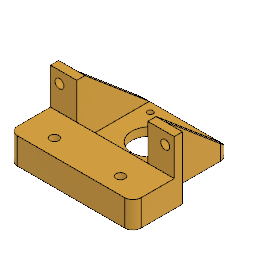
new2_elevated_Z_Motor_Mount v15 (Autodesk Fusion 360 design; units mm, degrees)
Autodesk Fusion 360 part; units mm, degrees
sketch "Sketch14" plane through (0, 0, 0) normal (0, 0, 1) x (1, 0, 0)
  line L0 (-37.5, 21) -> (37.5, 21)
  line L1 (37.5, 21) -> (37.5, -48)
  line L2 (37.5, -48) -> (-37.5, -48)
  line L3 (-37.5, -48) -> (-37.5, 21)
  line L4 (0, 21) -> (0, -48) construction
  circle A0 centre (0, 0) radius 11.2
  line L5 (15.5, 15.5) -> (-15.5, 15.5) construction
  line L6 (-15.5, 15.5) -> (-15.5, -15.5) construction
  line L7 (-15.5, -15.5) -> (15.5, -15.5) construction
  line L8 (15.5, -15.5) -> (15.5, 15.5) construction
  line L9 (15.5, 15.5) -> (-15.5, -15.5) construction
  line L10 (-15.5, 15.5) -> (15.5, -15.5) construction
  circle A1 centre (15.5, -15.5) radius 1.7
  circle A2 centre (15.5, 15.5) radius 1.7
  line L11 (-37.5, -38) -> (37.5, -38) construction
  circle A3 centre (20, -38) radius 5.5
  line L12 (26.5, 21) -> (26.5, -18)
  line L13 (26.5, -18) -> (37.5, -18)
  line L14 (-26.5, 21) -> (-26.5, -18)
  line L15 (-26.5, -18) -> (-37.5, -18)
  circle A4 centre (-20, -38) radius 5.5
  circle A5 centre (-15.5, 15.5) radius 1.7
  circle A6 centre (-15.5, -15.5) radius 1.7
  line L16 (-26.5, -18) -> (26.5, -18)
  line L17 (-37.5, -23) -> (37.5, -23)
  line L18 (21.5, 21) -> (21.5, -18)
  line L19 (-21.5, 21) -> (-21.5, -18)
  circle A7 centre (20, -38) radius 2.7
  circle A8 centre (-20, -38) radius 2.7
  line L20 (21.5, -18) -> (21.5, -23)
  line L21 (-21.5, -18) -> (-21.5, -23)
  dimension "d71" = 75
  dimension "d72" = 21
  dimension "d73" = 22.4
  dimension "d76" = 3.4
  dimension "d77" = 3.4
  dimension "d81" = 11
  dimension "d82" = 10
  dimension "d84" = 20
  dimension "d85" = 11
  dimension "d87" = 5
  dimension "d88" = 5
  dimension "d89" = 5.4
  dimension "d121" = 18
  dimension "d123" = 15
  dimension "d126" = 15.5
  dimension "d127" = 15.5
  constraint horizontal L0
  constraint vertical L1
  constraint horizontal L2
  constraint vertical L3
  constraint midpoint L0 L4.start
  constraint midpoint L2 L4.end
  constraint coincident A0.centre L4
  constraint coincident A0.centre origin
  constraint horizontal L5
  constraint perpendicular L5 L6
  constraint parallel L5 L7
  constraint parallel L6 L8
  constraint coincident L9 A0.centre
  constraint coincident L10 A0.centre
  constraint coincident L7.end L8.start
  constraint coincident L5.start L8.end
  constraint coincident L3 L11.start
  constraint coincident L1 L11.end
  constraint perpendicular L1 L11
  constraint coincident L11 A3.centre
  constraint coincident L0 L12.start
  constraint perpendicular L0 L12
  constraint coincident L1 L13.end
  constraint perpendicular L1 L13
  constraint symmetric L4 A1 A6
  constraint symmetric L4 A2 A5
  constraint symmetric L4 A3 A4
  constraint symmetric L4 L12.start L14.start
  constraint symmetric L4 L12.end L14.end
  constraint symmetric L4 L13.end L15.end
  constraint coincident L3 L17.start
  constraint coincident L1 L17.end
  constraint perpendicular L1 L17
  constraint coincident L0 L18.start
  constraint coincident L16 L18.end
  constraint perpendicular L16 L18
  constraint symmetric L4 L18.start L19.start
  constraint symmetric L4 L18.end L19.end
  constraint concentric A3 A7
  constraint symmetric L4 A7 A8
  constraint coincident L17 L20.end
  constraint perpendicular L17 L20
  constraint coincident L17 L21.end
  constraint perpendicular L17 L21
  measures "d71" distance of L0.start L0.end
  measures "d72" distance of A0.centre L0
  measures "d73" diameter of A0
  measures "d76" diameter of A1
  measures "d77" diameter of A2
  measures "d81" diameter of A3
  measures "d82" distance of L2 L11
  measures "d84" distance of L4 A3.centre
  measures "d85" distance of L12.end L13.end
  measures "d87" distance of L16 L17
  measures "d88" distance of L12 L18
  measures "d89" diameter of A7
  measures "d121" distance of A0.centre L16
  measures "d123" distance of L11 L17
  measures "d126" horizontal distance of A0.centre L5.end
  measures "d127" vertical distance of A0.centre L5.end
extrude "Extrude17" add sketch "Sketch14" along normal blind 5 contours L0 L14 L16 L19 | L3 L15 L16 L17 L21 | L0 L16 L18 L19 | L1 L2 L3 L17 | L0 L12 L16 L18 | L16 L17 L20 L21 | L1 L13 L16 L17 L20 | A3 | A4 makes body 1
extrude "Extrude18" add sketch "Sketch14" along normal blind 16 contours L1 L2 L3 L17 | A3 | A4 bodies 1
ref_plane "WorkPlane1" through (0, -35.5, 38) normal (0, 0, 1) x (1, 0, 0)
extrude "Extrude20" add sketch "Sketch14" along normal up to surface (38 mm away) contours L0 L14 L16 L19 | L3 L15 L16 L17 L21 | L0 L12 L16 L18 | L1 L13 L16 L17 L20 bodies 1
sketch "Sketch15" plane through (-26.5, 0, 0) normal (-1, 0, 0) x (0, -1, 0)
  line L0 (-21, 0) -> (18, 0)
  line L1 (18, 0) -> (18, 38)
  line L2 (18, 38) -> (-21, 38)
  line L3 (-21, 38) -> (-21, 0)
  line L4 (23, 5) -> (-21, 5)
  line L5 (-21, 5) -> (18, 38)
  constraint coincident L4.end L5.start
  constraint coincident L1.end L2.start
extrude "Extrude21" cut sketch "Sketch15" against normal through all contours L2 L3 L5 bodies 1
extrude "Extrude22" cut sketch "Sketch14" along normal up to surface (11 mm away) contours A3 | A4 bodies 1
extrude "Extrude23" add sketch "Sketch14" along normal blind 0.2 from surface at 11 contours A7 | A8 bodies 1
fillet "Fillet3" radius 5 4 edges at (26.5, 21, 2.5) (-26.5, 21, 2.5) (37.5, -48, 8) (-37.5, -48, 8) on bodies 1
sketch "Sketch16" plane through (0, -18, 0) normal (0, 1, 0) x (-1, 0, 0)
  line L0 (26.5, 0) -> (37.5, 0)
  line L1 (37.5, 0) -> (37.5, 38)
  line L2 (37.5, 38) -> (26.5, 38)
  line L3 (26.5, 38) -> (26.5, 0)
  line L4 (-37.5, 0) -> (-26.5, 0)
  line L5 (-26.5, 0) -> (-26.5, 38)
  line L6 (-26.5, 38) -> (-37.5, 38)
  line L7 (-37.5, 38) -> (-37.5, 0)
  line L8 (32, 38) -> (32, 0) construction
  line L9 (-32, 38) -> (-32, 0) construction
  line L10 (-37.5, 31) -> (37.5, 31) construction
  circle A0 centre (32, 31) radius 2.7
  circle A1 centre (-32, 31) radius 2.7
  line L11 (21.5, 16) -> (37.5, 16)
  dimension "d108" = 5.4
  dimension "d109" = 5.4
  dimension "d136" = 15
  constraint midpoint L2 L8.start
  constraint midpoint L0 L8.end
  constraint midpoint L6 L9.start
  constraint midpoint L4 L9.end
  constraint coincident L7 L10.start
  constraint coincident L1 L10.end
  constraint perpendicular L1 L10
  constraint coincident L8 A0.centre
  constraint coincident L10 A0.centre
  constraint coincident L10 A1.centre
  constraint coincident L9 A1.centre
  measures "d108" diameter of A0
  measures "d109" diameter of A1
  measures "d136" distance of A0.centre L11
extrude "Extrude24" cut sketch "Sketch16" against normal through all contours A0 | A1 bodies 1
ref_plane "WorkPlane2" through (0, -35.5, 46) normal (0, 0, 1) x (1, 0, 0)
extrude "Extrude26" add 1 faces at (4.8833, -20.9907, 5) along direction (0, 0, 1) blind 39 separate body on bodies 1 makes body 2
sketch "Sketch18" plane through (21.5, 0, 0) normal (1, 0, 0) x (0, 1, 0)
  line L0 (-23, 5) -> (21, 5)
  line L1 (21, 5) -> (21, 44)
  line L2 (21, 44) -> (-23, 44)
  line L3 (-23, 44) -> (-23, 5)
  line L4 (0, 0) -> (0, 44) construction
  line L5 (-8, 44) -> (8, 44)
  line L6 (8, 44) -> (8, 33)
  line L7 (8, 33) -> (-8, 33)
  line L8 (-8, 33) -> (-8, 44)
  point P0 (0, 33)
  dimension "d131" = 11
  dimension "d132" = 16
  dimension "d133" = 33
  constraint coincident L4.start origin
  constraint coincident L2 L4.end
  constraint perpendicular L2 L4
  constraint horizontal L5
  constraint vertical L6
  constraint horizontal L7
  constraint vertical L8
  constraint midpoint L7 P0
  constraint coincident L4 P0
  measures "d131" distance of L5.end L6.end
  measures "d132" distance of L5.start L5.end
  measures "d133" distance of L4.start L7
extrude "Extrude27" add sketch "Sketch18" along normal blind 7 contours L2 L5 L6 L7 L8 bodies 2
hidden bodies 2
equation "d77 = d76"
equation "d92 = 23 mm - 7 mm"
equation "d109 = d108"
named bodies: "Main", "Stepper"
